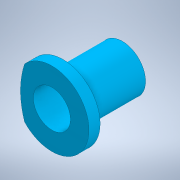
# Autodesk Inventor part: insertToScope
Saved by Autodesk Inventor 2022.1 (Build 261234020, 234B)
## iProperties
Created: 2020-09-09
Part Number: insertToScope
Material: PET Plastic
Document SubType Name: Modeling
Designer: robst
Density: 1.541 g/cm^3
Appearance: Sky Blue Medium
Author: robst
Autodesk Inventor part; units mm, degrees
ref_plane "YZ Plane" through (0, 0, 0) normal (1, 0, 0) x (0, 1, 0)
ref_plane "XZ Plane" through (0, 0, 0) normal (0, 1, 0) x (-1, 0, 0)
ref_plane "XY Plane" through (0, 0, 0) normal (0, 0, 1) x (1, 0, 0)
sketch "Sketch1" plane through (0, 0, 0) normal (0, 0, 1) x (1, 0, 0)
  circle A0 centre (0, 0) radius 15.875
  circle A1 centre (0, 0) radius 12.7
  dimension "d0" = 31.75
  dimension "d1" = 25.4
  constraints: 2 centre point, 2 coincident
  measures "d0" diameter of A0
  measures "d1" diameter of A1
extrude "Eyepiece Extrusion" add sketch "Sketch1" against normal blind 40.64
sketch "Sketch2" plane through (0, 0, 0) normal (0, 0, 1) x (1, 0, 0)
  circle A0 centre (0, 0) radius 12.7
  circle A1 centre (0, 0) radius 25.4
  dimension "d6" = 25.4
  dimension "d7" = 50.8
  constraints: 2 centre point, 2 coincident
  measures "d6" diameter of A0
  measures "d7" diameter of A1
extrude "Bolt Extrusion" add sketch "Sketch2" along normal blind 7.62
sketch "Sketch3" plane through (0, 0, 0) normal (0, 0, -1) x (-1, 0, 0)
  circle A0 centre (0, 0) radius 25.4 projected
  circle A1 centre (-33.1656, 0) radius 54.6286 projected
  circle A2 centre (0, 0) radius 12.7 projected
  circle A3 centre (0, 0) radius 15.875 projected
  arc A4 (18.442, -17.4658) -> (18.442, 17.4658) centre (-33.1656, 0) ccw
  circle A5 centre (0, 0) radius 25.4 construction
  point P0 (18.6815, 17.2093)
  point P1 (18.6815, -17.2093)
  dimension "d8" = 108.966
  constraints: 4 point on circle, 2 centre point, 2 coincident
  measures "d8" diameter of A4
extrude "Cutout For Filter Wheel" cut sketch "Sketch3" against normal through all contours A0 A1 picked at (23.8284, 2.0794)
sketch "Sketch7" plane through (0, 0, 0) normal (0, 0, -1) x (-1, 0, 0)
  arc A0 (18.6815, 17.2093) -> (18.6815, -17.2093) centre (0, 0) ccw projected
  circle A1 centre (-22.86, 0) radius 1.905 projected
  circle A2 centre (-10.16, -17.5976) radius 1.905 projected
  circle A3 centre (10.16, -17.5976) radius 1.905 projected
  arc A4 (21.4413, 1.54) -> (21.4413, -1.54) centre (20.32, 0) ccw projected
  circle A5 centre (10.16, 17.5976) radius 1.905 projected
  circle A6 centre (-10.16, 17.5976) radius 1.905 projected
  circle A7 centre (-20.32, 0) radius 1.905 projected
  point P0 (-11.43, -19.7973)
  point P1 (11.43, -19.7973)
  point P2 (22.86, 0)
  point P3 (11.43, 19.7973)
  point P4 (-11.43, 19.7973)
  dimension "d25" = 360
  dimension "d41" = 22.86
  constraints: 1 coincident, 7 other
  measures "d41" distance of A1.centre point (0, 0)
hole "Hole3" at (20.32, 0, 0) at (10.16, 17.5976, 0) at (-10.16, 17.5976, 0) at (-20.32, 0, 0) at (-11.43, -19.7973, 0) at (10.16, -17.5976, 0) direction (0, 0, 1) diameter 4.699 depth 7.1374 counterbore diameter 5.5372 counterbore depth 5.5524
equation "\"d0\" = outsideDiameter"
equation "\"d1\" = insideDiameter"
equation "\"d2\" = extrusionNoseDepth"
equation "\"d6\" = insideDiameter"
equation "\"d7\" = maxOutsideDiameter"
equation "\"d4\" = support"
equation "\"outsideDiameter\" = 31.75"
equation "\"insideDiameter\" = 25.4"
equation "\"support\" = 7.62"
equation "\"totalHeight\" = 44.45"
equation "\"maxOutsideDiameter\" = 50.8"
equation "\"eyepieceNoseDepth\" = 38.1"
equation "\"baseDepth\" = 2.54"
equation "\"extrusionNoseDepth\" = eyepieceNoseDepth + baseDepth"
body "Solid1"
